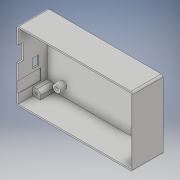
# Autodesk Inventor part: case_bottom
Saved by Autodesk Inventor 2019 (Build 230136000, 136)
## iProperties
Created: 2019-03-26
Part Number: case_bottom
Material: Generic
Document SubType Name: Modeling
Designer: janza
Density: 1 g/cm^3
Appearance: Default
Author: janza
## iProperties of the stored document case_bottom_3DPrint.ipt
Created: 2019-03-26
Part Number: case_bottom_3DPrint
Material: Generic
Document SubType Name: Modeling
Designer: janza
Density: 1 g/cm^3
Appearance: Default
Author: janza
Autodesk Inventor part; units mm, degrees
ref_plane "YZ Plane" through (0, 0, 0) normal (1, 0, 0) x (0, 1, 0)
ref_plane "XZ Plane" through (0, 0, 0) normal (0, 1, 0) x (-1, 0, 0)
ref_plane "XY Plane" through (0, 0, 0) normal (0, 0, 1) x (1, 0, 0)
sketch "zaklad" plane through (0, 0, 0) normal (0, 0, 1) x (1, 0, 0)
  line L0 (0, 0) -> (120, 0)
  line L1 (120, 0) -> (120, -70)
  line L2 (120, -70) -> (0, -70)
  line L3 (0, -70) -> (0, 0)
  dimension "d0" = 120
  dimension "d1" = 70
  constraints: 8 end point, 2 parallel, 1 horizontal, 1 perpendicular
  measures "d0" distance of L1.end L2.end
  measures "d1" distance of L0.end L1.end
extrude "Extrusion1" add sketch "zaklad" along normal blind 1.2 and the other way blind 0.4
sketch "uchyt_pro_desku" plane through (0, 0, 1.2) normal (0, 0, 1) x (1, 0, 0)
  line L0 (0, 0) -> (0, -70) projected
  line L1 (0, -35) -> (120, -35)
  line L2 (120, -70) -> (120, 0) projected
  circle A0 centre (17, -59) radius 4
  circle A1 centre (18, -11) radius 4
  circle A2 centre (92.5, -11) radius 4
  circle A3 centre (99, -59) radius 4
  dimension "d4" = 8
  dimension "d5" = 17
  dimension "d6" = 24
  dimension "d8" = 8
  dimension "d9" = 74.5
  dimension "d11" = 8
  dimension "d12" = 82
  dimension "d73" = 18
  constraints: 4 centre point, 2 end point, 2 midpoint
  measures "d4" diameter of A0
  measures "d5" distance from line of L0 A0.centre
  measures "d6" distance from line of L1 A0.centre
  measures "d8" diameter of A2
  measures "d9" distance of A2.centre A1.centre
  measures "d11" diameter of A3
  measures "d12" distance of A0.centre A3.centre
  measures "d73" distance from line of L0 A1.centre
extrude "Extrusion2" add sketch "uchyt_pro_desku" along normal blind 7
sketch "stena_RJ45" plane through (0, 0, 1.2) normal (0, 0, 1) x (1, 0, 0)
  line L0 (-1.6, -15.7) -> (0, -15.7)
  line L1 (0, -15.7) -> (0, -32.5)
  line L2 (0, -32.5) -> (-1.6, -32.5)
  line L3 (-1.6, -32.5) -> (-1.6, -15.7)
  circle A0 centre (18, -11) radius 4 projected
  line L4 (0, 0) -> (0, -70) projected
  dimension "d17" = 1.6
  dimension "d18" = 16.8
  dimension "d19" = 4.7
  dimension "d20" = 0
  constraints: 8 end point, 2 parallel, 1 coincident, 1 horizontal, 1 perpendicular
  measures "d17" distance of L1.end L2.end
  measures "d18" distance of L0.end L1.end
  measures "d19" distance from line of A0.centre L0
  measures "d20" distance between parallel lines of L4 L1
sketch "srouby_upevneni" plane through (0, 0, 1.2) normal (0, 0, 1) x (1, 0, 0)
  arc A0 (8, -66) -> (4, -62) centre (4, -66) ccw
  line L0 (0, -70) -> (120, -70) projected
  line L1 (0, 0) -> (0, -70) projected
  line L2 (8, -66) -> (8, -70)
  line L3 (4, -62) -> (0, -62)
  line L4 (0, -62) -> (0, -70)
  line L5 (8, -70) -> (0, -70)
  line L6 (120, -70) -> (120, 0) projected
  line L7 (120, -35) -> (0, -35)
  line L8 (60, -35) -> (60, -22.3833)
  arc A1 (4, -8) -> (8, -4) centre (4, -4) ccw
  line L9 (8, -4) -> (8, 0)
  line L10 (4, -8) -> (0, -8)
  line L11 (0, -8) -> (0, 0)
  line L12 (8, 0) -> (0, 0)
  arc A2 (116, -62) -> (112, -66) centre (116, -66) ccw
  line L13 (112, -66) -> (112, -70)
  line L14 (116, -62) -> (120, -62)
  line L15 (120, -62) -> (120, -70)
  line L16 (112, -70) -> (120, -70)
  line L17 (112, -4) -> (112, 0)
  arc A3 (112, -4) -> (116, -8) centre (116, -4) ccw
  line L18 (116, -8) -> (120, -8)
  line L19 (120, -8) -> (120, 0)
  line L20 (112, 0) -> (120, 0)
  dimension "d21" = 8
  constraints: 36 end point, 15 symmetric about line, 8 point on circle, 4 centre point, 4 tangent, 3 midpoint, 3 perpendicular, 2 point on line, 1 collinear, 1 vertical, 3 other
  measures "d21" diameter of A0
sketch "steny" plane through (0, 0, 1.2) normal (0, 0, 1) x (1, 0, 0)
  line L0 (0, -70) -> (120, -70) projected
  line L1 (120, -70) -> (120, 0) projected
  line L2 (120, 0) -> (0, 0) projected
  line L3 (0, 0) -> (0, -70) projected
  line L4 (0, -70) -> (0, -32.5)
  line L5 (0, -15.7) -> (0, 0)
  line L6 (0, -32.5) -> (-1.6, -32.5) projected
  line L7 (-1.6, -15.7) -> (0, -15.7) projected
  line L8 (-1.6, 1.6) -> (121.6, 1.6)
  line L9 (121.6, 1.6) -> (121.6, -71.6)
  line L10 (121.6, -71.6) -> (-1.6, -71.6)
  line L11 (-1.6, -71.6) -> (-1.6, -32.5)
  line L12 (-1.6, -15.7) -> (-1.6, 1.6)
  dimension "d74" = 1.6
  constraints: 16 end point, 2 collinear, 2 other
  measures "d74" distance between parallel lines of L2 L8
extrude "Extrusion3" add sketch "steny" along normal blind 30.5 and the other way blind 1.6 contours L0 L1 L2 L3 L7 L12 L8 L9 L10 L11 L6
extrude "Extrusion4" add sketch "stena_RJ45" along normal blind 25.5 and the other way blind 1.6 contours L0 L1 L2 L3
extrude "Extrusion5" add sketch "srouby_upevneni" along normal blind 15 contours L2 L0 L1 L3 A0 | L13 A2 L14 L6 L0 | L12 L9 A1 L10 L1 | L18 A3 L17 L20 L6
sketch "diry" plane through (0, 0, 1.2) normal (0, 0, 1) x (1, 0, 0)
  arc A0 (8, -66) -> (4, -62) centre (4, -66) ccw projected
  arc A1 (4, -8) -> (8, -4) centre (4, -4) ccw projected
  arc A2 (112, -4) -> (116, -8) centre (116, -4) ccw projected
  arc A3 (116, -62) -> (112, -66) centre (116, -66) ccw projected
  constraints: 5 coincident
hole "Hole1" at (116, -66, 1.2) at (116, -4, 1.2) at (4, -4, 1.2) at (4, -66, 1.2) direction (0, 0, -1) diameter 2.6 end through all both
sketch "uchyt_pro_desku_diry" plane through (99, -59, 8.2) normal (0, 0, 1) x (1, 0, 0)
  circle A0 centre (0, 0) radius 4 projected
  circle A1 centre (-82, 0) radius 4 projected
  circle A2 centre (-81, 48) radius 4 projected
  circle A3 centre (-6.5, 48) radius 4 projected
  point P0 (-99, 59)
  constraints: 4 coincident
hole "Hole2" at (99, -59, 8.2) at (17, -59, 8.2) at (18, -11, 8.2) at (92.5, -11, 8.2) direction (0, 0, -1) diameter 3.5 depth 7 countersink diameter 3.85 countersink angle 10
sketch "dira_USB" plane through (-1.6, -71.9, -0.4) normal (-1, 0, 0) x (0, 0, 1)
  line L0 (16.6, 36.7) -> (10.6, 36.7)
  line L1 (10.6, 36.7) -> (10.6, 26.7)
  line L2 (10.6, 26.7) -> (16.6, 26.7)
  line L3 (16.6, 26.7) -> (16.6, 36.7)
  line L4 (27.1, 39.4) -> (32.1, 39.4) projected
  line L5 (0, 0.3) -> (0, 73.5) projected
  point P0 (0.4, 71.9)
  point P1 (0, 0)
  point P2 (0, 73.8)
  dimension "d60" = 6
  dimension "d61" = 10
  dimension "d62" = 2.7
  dimension "d63" = 10.6
  constraints: 8 end point, 2 parallel, 1 horizontal, 1 perpendicular
  measures "d60" distance of L2.end L1.end
  measures "d61" distance of L1.end L0.end
  measures "d62" distance between parallel lines of L0 L4
  measures "d63" distance between parallel lines of L5 L1
extrude "Extrusion7" cut sketch "dira_USB" against normal blind 2
sketch "vyrez_napajeci_jack_nepouzivany" plane through (0, -70, 31.7) normal (1, 0, 0) x (0, 0, -1)
  line L0 (23.5, 21.8) -> (-6.5, 21.8)
  line L1 (-6.5, 21.8) -> (-6.5, 9.8)
  line L2 (-6.5, 9.8) -> (23.5, 9.8)
  line L3 (23.5, 9.8) -> (23.5, 21.8)
  line L4 (30.5, 62) -> (30.5, 8) projected
  line L5 (21.5, 24.8) -> (15.5, 24.8) projected
  point P0 (31.7, 70)
  dimension "d66" = 30
  dimension "d67" = 12
  dimension "d68" = 7
  dimension "d69" = 3
  constraints: 8 end point, 2 parallel, 1 horizontal, 1 perpendicular
  measures "d66" distance of L2.end L1.end
  measures "d67" distance of L1.end L0.end
  measures "d68" distance between parallel lines of L4 L3
  measures "d69" distance between parallel lines of L5 L0
extrude "Extrusion8" cut sketch "vyrez_napajeci_jack_nepouzivany" against normal blind 0.5
fillet "Fillet1" radius 2 4 edges at (-1.6, -71.6, 15.65) (-1.6, 1.6, 15.65) (121.6, -71.6, 15.65) (121.6, 1.6, 15.65)
body "Solid1"
